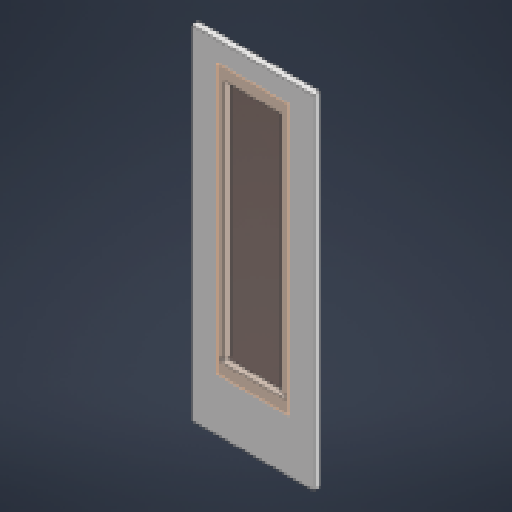
# Autodesk Inventor part: holderV2
Saved by Autodesk Inventor 2024.3 (Build 283343000, 343)
## iProperties
Created: 2025-08-18
Part Number: holderV2
Material: Generic
Document SubType Name: Modeling
Designer: giuseppe
Density: 1 g/cm^3
Appearance: Default
Author: giuseppe
Autodesk Inventor part; units mm, degrees
ref_plane "YZ Plane" through (0, 0, 0) normal (1, 0, 0) x (0, 1, 0)
ref_plane "XZ Plane" through (0, 0, 0) normal (0, 1, 0) x (-1, 0, 0)
ref_plane "XY Plane" through (0, 0, 0) normal (0, 0, 1) x (1, 0, 0)
ref_plane "Work Plane1" through (0, 0, 0) normal (0, 0, 1) x (1, 0, 0)
sketch "Sketch1" plane through (0, 0, 0) normal (0, 0, 1) x (1, 0, 0)
  line L0 (17.3205, 0) -> (17.3205, 60) projected
  line L1 (0, 60) -> (17.3205, 60) projected
  line L2 (0, 0) -> (0, 60) projected
  line L3 (0, 0) -> (0, -13.8) projected
  line L4 (-1.3617, -13.8) -> (0, -13.8) projected
  line L5 (-1.3617, -15) -> (-1.3617, -13.8) projected
  line L6 (18.6822, -15) -> (-1.3617, -15) projected
  line L7 (18.6822, -13.8) -> (18.6822, -15) projected
  line L8 (17.3205, -13.8) -> (18.6822, -13.8) projected
  line L9 (17.3205, 0) -> (17.3205, -13.8) projected
  line L10 (27.3205, 70) -> (-10, 70)
  line L11 (-10, 70) -> (-10, -35)
  line L12 (-10, -35) -> (27.3205, -35)
  line L13 (27.3205, -35) -> (27.3205, 70)
  dimension "d0" = 10
  dimension "d1" = 20
  dimension "d2" = 10
  dimension "d3" = 10
  constraints: 8 end point, 2 parallel, 1 horizontal, 1 perpendicular
  measures "d0" distance between parallel lines of L10 L1
  measures "d1" distance between parallel lines of L12 L6
  measures "d2" distance between parallel lines of L11 L2
  measures "d3" distance between parallel lines of L0 L13
extrude "Extrusion1" add sketch "Sketch1" against normal blind 2
body "Solid1"
